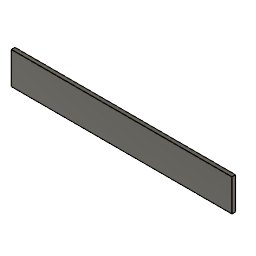
Template Base Plate (Autodesk Fusion 360 design; units mm, degrees)
part number: 2025-05-11-16-17-08-124
Autodesk Fusion 360 part; units mm, degrees
sketch "Sketch1" plane through (0, 0, 0) normal (0, 0, 1) x (1, 0, 0)
  line L0 (120, 20) -> (-120, 20)
  line L1 (-120, 20) -> (-120, -20)
  line L2 (-120, -20) -> (120, -20)
  line L3 (120, -20) -> (120, 20)
  line L4 (120, 20) -> (-120, -20) construction
  line L5 (-120, 20) -> (120, -20) construction
  dimension "d1" = 240
  dimension "d2" = 40
  constraint horizontal L0
  constraint perpendicular L0 L1
  constraint parallel L0 L2
  constraint parallel L1 L3
  constraint coincident L4 origin
  constraint coincident L5 origin
  measures "d1" distance of L1.end L2.end
  measures "d2" distance of L0.end L1.end
extrude "Extrude1" add sketch "Sketch1" along normal blind 5
sketch "Sketch2" plane through (0, 0, 5) normal (0, 0, 1) x (-1, 0, 0)
  line L0 (-120, 20) -> (-120, -20)
  line L1 (120, -20) -> (120, 20)
  line L2 (120, 20) -> (-120, 20)
  line L3 (120, -20) -> (-120, -20)
  line L4 (-120, -20) -> (-120, -16)
  line L5 (-120, -16) -> (120, -16)
  line L6 (120, -16) -> (120, -20)
  line L7 (-120, -20) -> (120, -20)
  dimension "d7" = 4
  constraint horizontal L3
  constraint vertical L4
  constraint horizontal L5
  constraint vertical L6
  constraint coincident L1.start L3.start
  measures "d7" distance of L1.start L5.end
extrude "Extrude3" add sketch "Sketch2" along normal blind 30 contours L0 L1 L3 L4 L5 L6 L7
sketch "Sketch3" plane through (0, 20, 0) normal (0, 1, 0) x (-1, 0, 0)
  line L0 (-120, 0) -> (120, 0)
  line L1 (120, 0) -> (120, 35)
  line L2 (120, 35) -> (-120, 35)
  line L3 (-120, 35) -> (-120, 0)
  line L4 (0, 35) -> (0, 0) construction
  line L5 (20.55, 35) -> (20.55, 0) construction
  line L6 (61.65, 35) -> (61.65, 0) construction
  line L7 (102.75, 35) -> (102.75, 0) construction
  line L8 (-20.55, 35) -> (-20.55, 0) construction
  line L9 (-61.65, 35) -> (-61.65, 0) construction
  line L10 (-102.75, 35) -> (-102.75, 0) construction
  line L11 (120, 17.5) -> (-120, 17.5) construction
  line L12 (27.95, 17.5) -> (24.25, 23.9086)
  line L13 (24.25, 23.9086) -> (16.85, 23.9086)
  line L14 (16.85, 23.9086) -> (13.15, 17.5)
  line L15 (13.15, 17.5) -> (16.85, 11.0914)
  line L16 (16.85, 11.0914) -> (24.25, 11.0914)
  line L17 (24.25, 11.0914) -> (27.95, 17.5)
  line L18 (-13.15, 17.5) -> (-16.85, 23.9086)
  line L19 (-16.85, 23.9086) -> (-24.25, 23.9086)
  line L20 (-24.25, 23.9086) -> (-27.95, 17.5)
  line L21 (-27.95, 17.5) -> (-24.25, 11.0914)
  line L22 (-24.25, 11.0914) -> (-16.85, 11.0914)
  line L23 (-16.85, 11.0914) -> (-13.15, 17.5)
  line L24 (-95.35, 17.5) -> (-99.05, 23.9086)
  line L25 (-99.05, 23.9086) -> (-106.45, 23.9086)
  line L26 (-106.45, 23.9086) -> (-110.15, 17.5)
  line L27 (-110.15, 17.5) -> (-106.45, 11.0914)
  line L28 (-106.45, 11.0914) -> (-99.05, 11.0914)
  line L29 (-99.05, 11.0914) -> (-95.35, 17.5)
  line L30 (95.35, 17.5) -> (99.05, 11.0914)
  line L31 (99.05, 11.0914) -> (106.45, 11.0914)
  line L32 (106.45, 11.0914) -> (110.15, 17.5)
  line L33 (110.15, 17.5) -> (106.45, 23.9086)
  line L34 (106.45, 23.9086) -> (99.05, 23.9086)
  line L35 (99.05, 23.9086) -> (95.35, 17.5)
  point P0 (20.55, 17.5)
  point P1 (-20.55, 17.5)
  point P2 (-102.75, 17.5)
  point P3 (102.75, 17.5)
  dimension "d10" = 20.55
  dimension "d11" = 41.1
  dimension "d12" = 41.1
  dimension "d13" = 41.1
  dimension "d14" = 41.1
  dimension "d15" = 20.55
  dimension "d16" = 7.4
  dimension "d17" = 7.4
  dimension "d18" = 7.4
  dimension "d19" = 7.4
  constraint midpoint L2 L4.start
  constraint coincident L4.end origin
  constraint coincident L2 L5.start
  constraint coincident L0 L5.end
  constraint perpendicular L0 L5
  constraint coincident L2 L6.start
  constraint coincident L0 L6.end
  constraint perpendicular L0 L6
  constraint coincident L0 L7.end
  constraint perpendicular L0 L7
  constraint coincident L2 L8.start
  constraint coincident L0 L8.end
  constraint perpendicular L0 L8
  constraint coincident L2 L9.start
  constraint coincident L0 L9.end
  constraint perpendicular L0 L9
  constraint coincident L2 L10.start
  constraint coincident L0 L10.end
  constraint perpendicular L0 L10
  constraint midpoint L1 L11.start
  constraint midpoint L3 L11.end
  constraint midpoint L5 P0
  constraint midpoint L8 P1
  constraint midpoint L10 P2
  constraint coincident L11 L30.start
  constraint midpoint L7 P3
  measures "d10" distance of L4 L5
  measures "d11" distance of L5 L6
  measures "d12" distance of L6 L7
  measures "d13" distance of L9 L10
  measures "d14" distance of L8 L9
  measures "d15" distance of L4 L8
  measures "d16" distance of L12.start P0
  measures "d17" distance of L18.start P1
  measures "d18" distance of L24.start P2
  measures "d19" distance of L30.start P3
extrude "Extrude4" add sketch "Sketch3" along normal blind 10 contours L12 L13 L14 L15 L16 L17 | L18 L19 L20 L21 L22 L23 | L24 L25 L26 L27 L28 L29 | L30 L31 L32 L33 L34 L35
extrude "Extrude8" cut 1 faces at (-40, -20, 1.6667) along direction (0, 1, 0) up to surface (36 mm away)
chamfer "Chamfer15" distance 1.5 angle 45 24 edges at (102.75, 30, 23.9086) (108.3, 30, 20.7043) (108.3, 30, 14.2957) (97.2, 30, 20.7043) (97.2, 30, 14.2957) (102.75, 30, 11.0914) (20.55, 30, 23.9086) (26.1, 30, 20.7043) (26.1, 30, 14.2957) (15, 30, 20.7043) (15, 30, 14.2957) (20.55, 30, 11.0914) (-20.55, 30, 23.9086) (-15, 30, 20.7043) (-15, 30, 14.2957) (-26.1, 30, 20.7043) (-26.1, 30, 14.2957) (-20.55, 30, 11.0914) (-102.75, 30, 23.9086) (-97.2, 30, 20.7043) (-97.2, 30, 14.2957) (-108.3, 30, 20.7043) (-108.3, 30, 14.2957) (-102.75, 30, 11.0914)
fillet "Fillet3" radius 1.5 24 edges at (99.05, 24.25, 23.9086) (110.15, 24.25, 17.5) (106.45, 24.25, 23.9086) (106.45, 24.25, 11.0914) (16.85, 24.25, 23.9086) (24.25, 24.25, 23.9086) (27.95, 24.25, 17.5) (24.25, 24.25, 11.0914) (-24.25, 24.25, 23.9086) (-16.85, 24.25, 23.9086) (-13.15, 24.25, 17.5) (-16.85, 24.25, 11.0914) (-106.45, 24.25, 23.9086) (-99.05, 24.25, 23.9086) (-95.35, 24.25, 17.5) (-99.05, 24.25, 11.0914) (-110.15, 24.25, 17.5) (-106.45, 24.25, 11.0914) (-27.95, 24.25, 17.5) (-24.25, 24.25, 11.0914) (13.15, 24.25, 17.5) (16.85, 24.25, 11.0914) (95.35, 24.25, 17.5) (99.05, 24.25, 11.0914)
equation "d22 = ( 240 / 6 ) * 1 mm"
equation "d60 = ( 80.8 / 3 ) * 1 mm"
equation "d61 = ( 80.8 / 3 ) * 1 mm"
equation "d64 = ( 26.933 / 2 ) * 1 mm"
equation "d65 = ( 26.933 / 2 ) * 1 mm"
equation "d73 = ( 80.8 / 3 ) * 1 mm"
equation "d74 = ( 80.8 / 3 ) * 1 mm"
equation "d77 = ( 26.933 / 2 ) * 1 mm"
equation "d81 = ( 17.5 / 2 ) * 1 mm"
